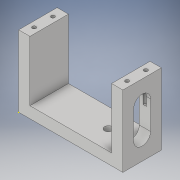
# Autodesk Inventor part: kreplenie2
Saved by Autodesk Inventor 2019 (Build 230136000, 136)
## iProperties
Created: 2019-09-02
Part Number: kreplenie2
Material: Типовые
Document SubType Name: Modeling
Designer: UlyaKZ
Density: 1 g/cm^3
Appearance: По умолчанию
Author: UlyaKZ
Autodesk Inventor part; units mm, degrees
ref_plane "YZ Plane" through (0, 0, 0) normal (1, 0, 0) x (0, 1, 0)
ref_plane "XZ Plane" through (0, 0, 0) normal (0, 1, 0) x (-1, 0, 0)
ref_plane "XY Plane" through (0, 0, 0) normal (0, 0, 1) x (1, 0, 0)
sketch "Эскиз1" plane through (0, 0, 0) normal (0, 0, 1) x (1, 0, 0)
  line L0 (0, 0) -> (55.5, 0)
  line L1 (55.5, 0) -> (55.5, 6)
  line L2 (55.5, 6) -> (0, 6)
  line L3 (0, 6) -> (0, 0)
  line L4 (0, 6) -> (6, 6)
  line L5 (6, 6) -> (6, 38)
  line L6 (6, 38) -> (0, 38)
  line L7 (0, 38) -> (0, 6)
  line L8 (55.5, 6) -> (49.5, 6)
  line L9 (49.5, 6) -> (49.5, 38)
  line L10 (49.5, 38) -> (55.5, 38)
  line L11 (55.5, 38) -> (55.5, 6)
  dimension "d0" = 38
  dimension "d1" = 6
  dimension "d2" = 6
  dimension "d3" = 6
  dimension "d4" = 38
  dimension "d5" = 55.5
  constraints: 24 end point, 6 parallel, 3 horizontal, 3 perpendicular
  measures "d0" distance between parallel lines of L0 L10
  measures "d1" distance between parallel lines of L0 L2
  measures "d2" distance between parallel lines of L11 L9
  measures "d3" distance between parallel lines of L5 L7
  measures "d4" distance between parallel lines of L0 L6
  measures "d5" distance between parallel lines of L3 L1
extrude "Выдавливание1" add sketch "Эскиз1" along normal blind 20.5
sketch "Эскиз2" plane through (55.5, 0, 0) normal (1, 0, 0) x (0, 0, -1)
  circle A0 centre (-10.25, 26.5) radius 4.5
  circle A1 centre (-10.25, 11.5) radius 4.5
  line L0 (-5.75, 26.5) -> (-5.75, 11.5)
  line L1 (-14.75, 26.5) -> (-14.75, 11.5)
  line L2 (0, 0) -> (-20.5, 0) projected
  point P0 (-10.25, 0)
  dimension "d8" = 9
  dimension "d9" = 11.5
  dimension "d10" = 24
  constraints: 4 end point, 4 point on circle, 3 tangent, 2 centre point, 2 vertical alignment, 1 equal radius, 1 midpoint, 1 parallel
  measures "d8" distance between parallel lines of L0 L1
  measures "d9" distance from line of L2 A1.centre
extrude "Выдавливание2" cut sketch "Эскиз2" against normal up to next
sketch "Эскиз3" plane through (0, 0, 0) normal (0, -1, 0) x (1, 0, 0)
  circle A0 centre (37.5, 10.25) radius 2
  line L0 (55.5, 0) -> (55.5, 20.5) projected
  point P0 (0, 0)
  point P1 (55.5, 10.25)
  dimension "d13" = 4
  dimension "d14" = 18
  constraints: 1 centre point, 1 horizontal alignment, 1 midpoint
  measures "d13" diameter of A0
  measures "d14" distance from line of L0 A0.centre
extrude "Выдавливание3" cut sketch "Эскиз3" against normal up to next
sketch "Эскиз4" plane through (49.5, 38, 0) normal (0, 1, 0) x (1, 0, 0)
  circle A0 centre (3, -15.25) radius 1
  circle A1 centre (3, -5.25) radius 1
  line L0 (0, 0) -> (0, -20.5) projected
  line L1 (6, -20.5) -> (0, -20.5) projected
  line L2 (3, -5.25) -> (3, -15.25) construction
  point P0 (-49.5, 0)
  point P1 (3, -10.25)
  point P2 (0, -10.25)
  dimension "d17" = 2
  dimension "d18" = 10
  dimension "d19" = 2
  constraints: 2 centre point, 2 end point, 2 midpoint, 1 equal radius, 1 horizontal alignment, 1 vertical, 1 vertical alignment
  measures "d17" diameter of A0
  measures "d18" distance of L2.start L2.end
  measures "d19" distance edge to line of A1 L0
extrude "Выдавливание4" cut sketch "Эскиз4" against normal blind 16
sketch "Эскиз5" plane through (0, 38, 0) normal (0, 1, 0) x (1, 0, 0)
  circle A0 centre (3, -5.25) radius 1
  circle A1 centre (3, -15.25) radius 1
  circle A2 centre (52.5, -5.25) radius 1 projected
  circle A3 centre (52.5, -15.25) radius 1 projected
  line L0 (6, 0) -> (0, 0) projected
  point P0 (3, 0)
  dimension "d23" = 2
  constraints: 2 centre point, 2 horizontal alignment, 2 vertical alignment, 1 equal radius, 1 midpoint
  measures "d23" diameter of A1
extrude "Выдавливание5" cut sketch "Эскиз5" against normal up to next contours A0 | A1
sketch "Эскиз6" plane through (0, 0, 20.5) normal (0, 0, 1) x (1, 0, 0)
  point P0 (0, 0)
